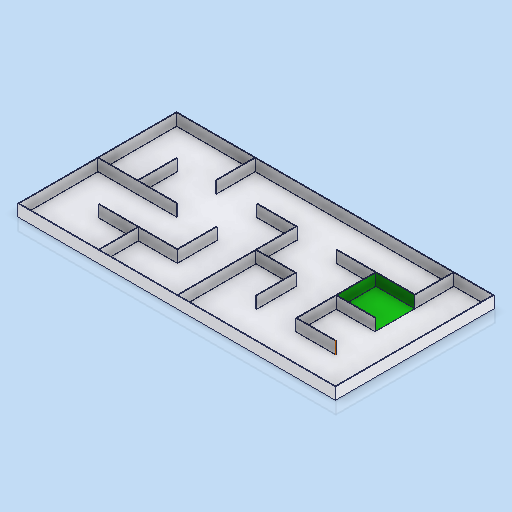
# Autodesk Inventor part: лабиринт
Saved by Autodesk Inventor 2025 (Build 290162000, 162)
## iProperties
Created: 2025-02-28
Part Number: лабиринт
Material: Типовые
Document SubType Name: Modeling
Designer: volko
Density: 1 g/cm^3
Appearance: PTFE
Author: volko
Autodesk Inventor part; units mm, degrees
ref_plane "YZ Plane" through (0, 0, 0) normal (1, 0, 0) x (0, 1, 0)
ref_plane "XZ Plane" through (0, 0, 0) normal (0, 1, 0) x (-1, 0, 0)
ref_plane "XY Plane" through (0, 0, 0) normal (0, 0, 1) x (1, 0, 0)
sketch "Эскиз1" plane through (0, 0, 0) normal (0, 1, 0) x (-1, 0, 0)
  line L0 (-4060, 2020) -> (-4060, -2020)
  line L1 (-3060, -2020) -> (-3060, -1020)
  line L2 (-2060, 1000) -> (-3060, 1000)
  line L3 (-2060, -20) -> (-3060, -20)
  line L4 (-5712, 0) -> (5712, 0) projected
  line L5 (5712, 0) -> (-5712, 0) projected
  line L6 (0, -2856) -> (0, 2856) projected
  line L7 (4080, 2040) -> (-4080, 2040)
  line L8 (-4080, 2040) -> (-4080, -2040)
  line L9 (-4080, -2040) -> (4080, -2040)
  line L10 (4080, -2040) -> (4080, 2040)
  line L11 (-3040, -2020) -> (-3040, -1040)
  line L12 (-3040, -1040) -> (-2040, -1040)
  line L13 (-2060, 0) -> (-3060, 0)
  line L14 (-3060, 1020) -> (-2040, 1020)
  line L15 (-2040, 1020) -> (-2040, -1020)
  line L16 (-3060, -1020) -> (-2060, -1020)
  line L17 (-2060, -1020) -> (-2060, -20)
  line L18 (-2060, 0) -> (-2060, 1000)
  line L19 (-3060, 1020) -> (-3060, 1000)
  line L20 (-3060, -20) -> (-3060, 0)
  line L21 (-20, -1040) -> (1000, -1040)
  line L22 (0, 2020) -> (0, -1020)
  line L23 (0, -1020) -> (1000, -1020)
  line L24 (1000, -1020) -> (1000, -1040)
  line L25 (-2040, -1020) -> (-1040, -1020)
  line L26 (-1040, -1020) -> (-1040, -1040)
  line L27 (-1040, -1040) -> (-2040, -1040)
  line L28 (-1040, 1020) -> (-1040, 0)
  line L29 (-1040, 0) -> (-20, 0)
  line L30 (-1020, 1020) -> (-1020, 20)
  line L31 (-20, 2020) -> (-20, 20)
  line L32 (-20, 0) -> (-20, -1040)
  line L33 (-1040, 1020) -> (-1020, 1020)
  line L34 (2040, -2020) -> (2040, -1020)
  line L35 (2040, -1020) -> (2060, -1020)
  line L36 (2060, -1020) -> (2060, -2020)
  line L37 (2000, 1020) -> (2000, 2020)
  line L38 (2020, 2020) -> (2020, 1020)
  line L39 (2000, 1020) -> (1000, 1020)
  line L40 (1000, 1020) -> (1000, 0)
  line L41 (1386.822, 1000) -> (1386.822, 997)
  line L42 (-20, 2020) -> (-4060, 2020)
  line L43 (4060, 2020) -> (2020, 2020)
  line L44 (2000, 2020) -> (0, 2020)
  line L45 (-20, 20) -> (-1020, 20)
  line L46 (4060, 0) -> (2040, 0)
  line L47 (2040, 0) -> (2040, -20)
  line L48 (2040, -20) -> (3040, -20)
  line L49 (3040, -20) -> (3040, -1020)
  line L50 (3040, -1020) -> (3060, -1020)
  line L51 (3060, -1020) -> (3060, -20)
  line L52 (3060, -20) -> (4060, -20)
  line L53 (4060, -2020) -> (4060, -20)
  line L54 (4060, 0) -> (4060, 2020)
  line L55 (-4060, -2020) -> (2040, -2020)
  line L56 (2060, -2020) -> (4060, -2020)
  line L57 (1000, 0) -> (1020, 0)
  line L58 (1020, 0) -> (1020, 1000)
  line L59 (1020, 1000) -> (3020, 1000)
  line L60 (3020, 1000) -> (3020, 1020)
  line L61 (2020, 1020) -> (3020, 1020)
  point P0 (0, 0)
  point P1 (4080, 0)
  point P2 (0, 2040)
  point P3 (1093.178, 0)
  point P4 (-20, 0)
  point P5 (0, 1020)
  point P6 (0, 2020)
  point P7 (-4060, 0)
  point P8 (0, 0)
  point P9 (9.9936, 474.3673)
  point P10 (-4080, 0)
  point P11 (0, -2040)
  point P12 (-1040, 0)
  point P13 (0, -2020)
  point P14 (0, -1020)
  point P15 (0, -1040)
  dimension "d6" = 20
  dimension "d10" = 1000
  dimension "d11" = 1000
  dimension "d17" = 20
  dimension "d18" = 20
  dimension "d20" = 20
  dimension "d21" = 20
  dimension "d22" = 20
  dimension "d23" = 1000
  dimension "d24" = 20
  dimension "d26" = 20
  dimension "d27" = 20
  dimension "d28" = 20
  dimension "d29" = 20
  dimension "d30" = 20
  dimension "d31" = 20
  dimension "d32" = 20
  dimension "d33" = 20
  dimension "d34" = 20
  dimension "d35" = 20
  constraints: 118 end point, 33 perpendicular, 17 collinear, 15 equal length, 11 parallel, 9 horizontal, 9 vertical, 7 point on line, 4 other
  measures "d6" distance between parallel lines of L1 L11
  measures "d10" distance between parallel lines of L13 L2
  measures "d11" distance of L1.start L1.end
  measures "d17" distance between parallel lines of L28 L30
  measures "d18" distance between parallel lines of L37 L38
  measures "d20" distance between parallel lines of L12 L16
  measures "d21" distance between parallel lines of L3 L4
  measures "d22" distance between parallel lines of L2 L14
  measures "d23" distance between parallel lines of L0 L1
  measures "d24" distance between parallel lines of L17 L15
  measures "d26" distance between parallel lines of L22 L32
  measures "d27" distance between parallel lines of L21 L23
  measures "d28" distance between parallel lines of L34 L36
  measures "d29" distance between parallel lines of L5 L45
  measures "d30" distance between parallel lines of L8 L0
  measures "d31" distance between parallel lines of L9 L55
  measures "d32" distance between parallel lines of L52 L46
  measures "d33" distance between parallel lines of L49 L51
  measures "d34" distance between parallel lines of L59 L61
  measures "d35" distance between parallel lines of L58 L40
extrude "Выдавливание1" add sketch "Эскиз1" along normal blind 300 contours L0 L4 L8 L7 L6 L28 L33 L30 L45 L31 L42 | L0 L55 L6 L9 L8 L4 | L4 L15 L25 L26 L27 L12 L11 L55 L1 L16 L17 L3 L20 | L18 L2 L19 L14 L15 L4 | L7 L10 L4 L54 L43 L38 L61 L60 L59 L58 L40 L39 L37 L44 L6 | L6 L55 L34 L35 L36 L56 L53 L52 L51 L50 L49 L48 L47 L4 L10 L9 | L21 L32 L4 L6 | L6 L23 L24 L21
extrude "Выдавливание2" add sketch "Эскиз1" against normal blind 10 contours L42 L31 L45 L30 L33 L28 L4 L15 L14 L19 L2 L18 L0 | L4 L20 L3 L17 L16 L1 L55 L0 | L11 L12 L27 L26 L25 L15 L4 L32 L21 L6 L55 | L6 L21 L24 L23 L4 L47 L48 L49 L50 L51 L52 L53 L56 L36 L35 L34 L55 | L44 L37 L39 L40 L4 L6 | L4 L58 L59 L60 L61 L38 L43 L54
ref_plane "РабПлоскость1" through (3060, 300, 1020) normal (1, 0, 0) x (0, 0, -1)
sketch "Эскиз2" plane through (0, 0, 0) normal (0, 1, 0) x (1, 0, 0)
  line L0 (3060, 20) -> (2060, 20) projected
  line L1 (3060, 20) -> (3060, 1024)
  line L2 (2060, 20) -> (2060, 1020) projected
  line L3 (2060, 1020) -> (3060, 1020) projected
  point P0 (0, 0)
  constraints: 2 end point, 1 vertical
extrude "Выдавливание3" add sketch "Эскиз2" against normal blind 10 separate body
equation "\"d10\" = d1"
equation "\"d20\" = d3"
equation "\"d21\" = d3"
equation "\"d22\" = d3"
equation "\"d23\" = d1"
equation "\"d24\" = d3"
equation "\"d26\" = d3"
equation "\"d27\" = d3"
equation "\"d28\" = d3"
equation "\"d29\" = d3"
equation "\"d30\" = d3"
equation "\"d31\" = d3"
equation "\"d32\" = d3"
equation "\"d33\" = d3"
equation "\"d34\" = d3"
equation "\"d35\" = d3"
equation "\"d1\" = 1000"
equation "\"d3\" = 20"
